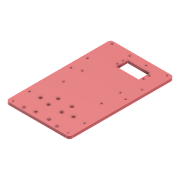
# Autodesk Inventor part: base plate
Saved by Autodesk Inventor 2022 (Build 260153000, 153)
## iProperties
Created: 2024-03-20
Part Number: base plate
Material: Generic
Document SubType Name: Modeling
Designer: david
Density: 1 g/cm^3
Appearance: Smooth - Red
Author: david
Autodesk Inventor part; units mm, degrees
ref_plane "YZ Plane" through (0, 0, 0) normal (1, 0, 0) x (0, 1, 0)
ref_plane "XZ Plane" through (0, 0, 0) normal (0, 1, 0) x (-1, 0, 0)
ref_plane "XY Plane" through (0, 0, 0) normal (0, 0, 1) x (1, 0, 0)
sketch "Sketch1" plane through (0, 0, 0) normal (0, 1, 0) x (-1, 0, 0)
  line L0 (57.5, -190) -> (57.5, -190) construction
  line L1 (-57.5, -190) -> (-57.5, 0) construction
  line L2 (-57.5, 0) -> (57.5, 0)
  line L3 (57.5, 0) -> (57.5, -190) construction
  line L4 (80.5, 0) -> (-80.5, 0) construction
  line L5 (0, -228) -> (0, 38) construction
  line L6 (57.5, -190) -> (-57.5, -190)
  line L7 (-57.5, -190) -> (-57.5, -190) construction
  line L8 (-57.5, 0) -> (57.5, 0)
  line L9 (57.5, 0) -> (57.5, -40)
  line L10 (57.5, -40) -> (-57.5, -40) construction
  line L11 (-57.5, -40) -> (-57.5, 0)
  line L12 (57.5, -40) -> (57.5, -190)
  line L13 (-57.5, -190) -> (-57.5, -40)
  point P0 (0, 0)
  dimension "width" = 115
  dimension "Length" = 190
  dimension "d2" = 115
  dimension "d92" = 40
  constraints: 24 end point, 6 parallel, 4 horizontal, 4 perpendicular, 1 collinear, 1 point on line, 1 symmetric about line, 1 vertical alignment, 1 other
  measures "width" distance of L1.end L2.end
  measures "Length" distance of L1.start L1.end
  measures "d2" distance of L6.end L0.end
  measures "d92" distance between parallel lines of L2 L10
extrude "Base" add sketch "Sketch1" against normal blind 5
sketch "Sketch2" plane through (0, 0, 0) normal (0, 1, 0) x (1, 0, 0)
  line L0 (30, 35) -> (50, 35) construction
  line L1 (50, 35) -> (50, 5) construction
  line L2 (50, 5) -> (30, 5) construction
  line L3 (30, 5) -> (30, 35) construction
  line L4 (0, 228) -> (0, -38) construction
  line L5 (-30, 35) -> (-50, 35) construction
  line L6 (-50, 35) -> (-50, 5) construction
  line L7 (-50, 5) -> (-30, 5) construction
  line L8 (-30, 5) -> (-30, 35) construction
  line L9 (-57.5, 0) -> (57.5, 0) projected
  line L10 (-35, 40) -> (-25, 40) construction
  line L11 (-25, 40) -> (-25, 0) construction
  line L12 (-25, 0) -> (-35, 0) construction
  line L13 (-35, 0) -> (-35, 40) construction
  line L14 (-30, 30) -> (-30, 10) construction
  line L15 (30, 5) -> (30, 35) construction
  line L16 (35, 40) -> (25, 40) construction
  line L17 (25, 40) -> (25, 0) construction
  line L18 (25, 0) -> (35, 0) construction
  line L19 (35, 0) -> (35, 40) construction
  line L20 (30, 30) -> (30, 10) construction
  point P0 (0, 0)
  point P1 (-30, 40)
  point P2 (-30, 20)
  point P3 (-25, 20)
  point P4 (-30, 20)
  point P5 (30, 40)
  point P6 (30, 20)
  point P7 (25, 20)
  point P8 (30, 20)
  dimension "d5" = 20
  dimension "d6" = 30
  dimension "d8" = 5
  dimension "d16" = 10
  dimension "d18" = 20
  dimension "d19" = 10
  dimension "d20" = 50
  constraints: 38 end point, 18 symmetric about line, 8 coincident, 4 midpoint, 4 parallel, 4 point on line, 2 horizontal, 2 perpendicular, 1 horizontal alignment, 1 vertical alignment
  measures "d5" distance of L1.end L2.end
  measures "d6" distance of L0.end L1.end
  measures "d8" distance between parallel lines of L9 L2
  measures "d16" distance of L10.start L10.end
  measures "d18" distance of L14.end L14.start
  measures "d19" vertical distance of L10.end L14.start
  measures "d20" distance between parallel lines of L17 L11
hole "Bearing Holder Mounting Holes" at (30, 0, -35) at (50, 0, -35) at (50, 0, -5) at (-50, 0, -5) at (-30, 0, -35) at (-50, 0, -35) at (-30, 0, -5) at (30, 0, -5) direction (0, -1, 0) diameter 3.4 end through all
fillet "Fillet1" radius 5 4 edges at (57.5, -2.5, 0) (57.5, -2.5, -190) (-57.5, -2.5, -190) (-57.5, -2.5, 0)
sketch "Sketch5" plane through (0, 0, 0) normal (0, 1, 0) x (1, 0, 0)
  line L0 (-34.5, 81.5) -> (34.5, 81.5) construction
  line L1 (34.5, 81.5) -> (34.5, 115.5) construction
  line L2 (34.5, 115.5) -> (-34.5, 115.5) construction
  line L3 (-34.5, 115.5) -> (-34.5, 81.5) construction
  line L4 (-57.5, 0) -> (52.5, 0) projected
  point P0 (0, 0)
  point P1 (-52.2987, 0)
  point P2 (0, 81.5)
  dimension "d41" = 34
  dimension "d42" = 69
  dimension "d43" = 81.5
  constraints: 8 end point, 2 parallel, 1 horizontal, 1 midpoint, 1 perpendicular, 1 vertical alignment
  measures "d41" distance of L2.end L0.start
  measures "d42" distance of L1.end L2.end
  measures "d43" distance between parallel lines of L4 L0
hole "12v Motor Mount Mounting Holes" at (-34.5, 0, -115.5) at (-34.5, 0, -81.5) at (34.5, 0, -81.5) at (34.5, 0, -115.5) direction (0, -1, 0) diameter 3.2 end through all
sketch "Sketch8" plane through (0, 0, 0) normal (0, 1, 0) x (1, 0, 0)
  line L0 (-10, 153.5) -> (30, 153.5)
  line L1 (30, 153.5) -> (30, 173.5)
  line L2 (30, 173.5) -> (-10, 173.5)
  line L3 (-10, 173.5) -> (-10, 153.5)
  line L4 (52.5, 190) -> (-52.5, 190) projected
  line L5 (-57.5, 0) -> (52.5, 0) projected
  point P0 (0, 0)
  point P1 (0, 190)
  dimension "d64" = 20
  dimension "d65" = 40
  dimension "d67" = 10
  dimension "d107" = 153.5
  constraints: 8 end point, 2 parallel, 1 horizontal, 1 midpoint, 1 perpendicular
  measures "d64" distance of L2.end L0.start
  measures "d65" distance of L1.end L2.end
  measures "d67" distance from line of point (0, 190) L3
  measures "d107" distance between parallel lines of L5 L0
extrude "Servo Cutout 2" cut sketch "Sketch8" against normal through all
sketch "Sketch9" plane through (0, 0, 0) normal (0, 1, 0) x (1, 0, 0)
  line L0 (-13.925, 158.5) -> (33.925, 158.5) construction
  line L1 (33.925, 158.5) -> (33.925, 168.5) construction
  line L2 (33.925, 168.5) -> (-13.925, 168.5) construction
  line L3 (-13.925, 168.5) -> (-13.925, 158.5) construction
  line L4 (30, 173.5) -> (30, 153.5) construction
  line L5 (-10, 153.5) -> (-10, 173.5) construction
  point P0 (0, 0)
  point P1 (-10, 163.5)
  point P2 (-13.925, 163.5)
  point P3 (-10, 163.5)
  dimension "d70" = 3.925
  dimension "d71" = 5
  dimension "d72" = 3.925
  constraints: 8 end point, 3 midpoint, 2 parallel, 1 horizontal, 1 horizontal alignment, 1 perpendicular
  measures "d70" distance between parallel lines of L1 L4
  measures "d71" vertical distance of L2.end point (-10, 163.5)
  measures "d72" distance between parallel lines of L5 L3
hole "Servo Mounting Holes 2" at (-13.925, 0, -158.5) at (-13.925, 0, -168.5) at (33.925, 0, -158.5) at (33.925, 0, -168.5) direction (0, -1, 0) diameter 3.4 end through all
sketch "Sketch10" plane through (0, 0, 0) normal (0, 1, 0) x (1, 0, 0)
  circle A0 centre (33.925, 158.5) radius 1.7 construction
  circle A1 centre (-13.925, 158.5) radius 1.7 construction
  circle A2 centre (-13.925, 168.5) radius 1.7 construction
  circle A3 centre (33.925, 168.5) radius 1.7 construction
  line L0 (-10, 153.5) -> (30, 153.5) construction
  line L1 (30, 153.5) -> (30, 173.5) construction
  line L2 (30, 173.5) -> (-10, 173.5) construction
  line L3 (-10, 173.5) -> (-10, 153.5) construction
  circle A4 centre (34.5, 81.5) radius 1.6 construction
  circle A5 centre (-34.5, 115.5) radius 1.6 construction
  circle A6 centre (-34.5, 81.5) radius 1.6 construction
  circle A7 centre (34.5, 115.5) radius 1.6 construction
  arc A8 (52.5, 0) -> (57.5, 5) centre (52.5, 5) ccw construction
  line L4 (52.5, 0) -> (-52.5, 0) construction
  line L5 (-57.5, 5) -> (-57.5, 185) construction
  line L6 (-52.5, 190) -> (52.5, 190) construction
  line L7 (57.5, 185) -> (57.5, 5) construction
  circle A9 centre (-30, 5) radius 1.7 construction
  circle A10 centre (-30, 35) radius 1.7 construction
  circle A11 centre (50, 5) radius 1.7 construction
  circle A12 centre (30, 35) radius 1.7 construction
  circle A13 centre (50, 35) radius 1.7 construction
  circle A14 centre (-50, 5) radius 1.7 construction
  circle A15 centre (-50, 35) radius 1.7 construction
  circle A16 centre (30, 5) radius 1.7 construction
  line L8 (0, 229.4046) -> (0, -39.4422) construction
  arc A17 (-52.5, 190) -> (-57.5, 185) centre (-52.5, 185) ccw projected
  arc A18 (57.5, 185) -> (52.5, 190) centre (52.5, 185) ccw projected
  arc A19 (-57.5, 5) -> (-52.5, 0) centre (-52.5, 5) ccw projected
  point P0 (-50, 185)
  point P1 (50, 185)
  dimension "d93" = 5
  dimension "d94" = 50
  dimension "d111" = 50
  constraints: 1 symmetric about line
  measures "d93" distance from line of L6 point (-50, 185)
  measures "d94" distance from line of L8 point (-50, 185)
  measures "d111" distance from line of A14.centre L8
hole "Extra Holes For Top Plate" at (-50, 0, -185) at (50, 0, -185) direction (0, -1, 0) diameter 3.4 depth 6
sketch "Sketch11" plane through (0, 0, 0) normal (0, 1, 0) x (1, 0, 0)
  line L0 (49.5, 140) -> (49.5, 110) construction
  line L1 (52.5, 190) -> (-52.5, 190) construction
  line L2 (0, 228) -> (0, -38) projected
  line L3 (-49.5, 140) -> (-49.5, 110) construction
  line L4 (15, 182) -> (-15, 182)
  line L5 (57.5, 5) -> (57.5, 185) projected
  point P0 (0, 0)
  point P1 (0, 182)
  point P2 (0, 190)
  dimension "d95" = 50
  dimension "d96" = 30
  dimension "d108" = 30
  dimension "d109" = 8
  dimension "d110" = 8
  constraints: 6 coincident, 6 end point, 4 symmetric about line, 2 midpoint, 1 horizontal, 1 parallel, 1 vertical alignment
  measures "d95" distance from line of L1 L0.start
  measures "d96" distance of L0.start L0.end
  measures "d108" distance of L4.start L4.end
  measures "d109" distance between parallel lines of L1 L4
  measures "d110" distance between parallel lines of L5 L0
hole "Ultrasonic Sensor Mounting Holes" at (49.5, 0, -140) at (49.5, 0, -110) at (-49.5, 0, -110) at (-49.5, 0, -140) at (-15, 0, -182) at (15, 0, -182) direction (0, -1, 0) diameter 3.4 depth 6
thicken "Thicken2" operation add thickness 0.45 both sides no extend neighbours yes toward (-1, 0, 0) faces at (-10, -1.6667, -166.8333) (16.6667, -3.3333, -173.5) (3.3333, -1.6667, -153.5) (30, -1.6667, -160.1667)
sketch "Sketch12" plane through (0, 0, 0) normal (0, 1, 0) x (1, 0, 0)
  circle A0 centre (30, 35) radius 1.7 construction
  circle A1 centre (30, 5) radius 1.7 construction
  line L0 (30, 35) -> (30, 5) construction
  line L1 (-12, 31.5) -> (12, 31.5)
  line L2 (12, 31.5) -> (12, 8.5)
  line L3 (12, 8.5) -> (-12, 8.5)
  line L4 (-12, 8.5) -> (-12, 31.5)
  line L5 (-12, 31.5) -> (12, 8.5) construction
  line L6 (12, 31.5) -> (-12, 8.5) construction
  point P0 (0, 0)
  point P1 (12, 20)
  point P2 (30, 20)
  point P3 (0, 8.5)
  point P4 (-12, 31.5)
  point P5 (12, 31.5)
  point P6 (0, 20)
  point P7 (0, 20)
  point P8 (0, 20)
  dimension "d121" = 23
  dimension "d122" = 24
  constraints: 14 end point, 5 midpoint, 2 coincident, 2 horizontal alignment, 2 parallel, 2 vertical alignment, 1 horizontal, 1 perpendicular, 1 vertical
  measures "d121" distance of L1.end L2.end
  measures "d122" distance of L1.start L1.end
hole "Differential Stopper Mounting Holes" at (-12, 0, -31.5) at (12, 0, -31.5) at (-12, 0, -8.5) at (12, 0, -8.5) direction (0, -1, 0) diameter 3.4 end through all counterbore diameter 6 counterbore depth 2
sketch "Sketch13" plane through (0, 0, 0) normal (0, -1, 0) x (1, 0, 0)
  line L0 (-12.5, -49.5) -> (12.5, -49.5)
  line L1 (52.5, 0) -> (-52.5, 0) projected
  point P0 (0, 0)
  point P1 (0, -49.5)
  point P2 (-57.5, 0)
  dimension "d123" = 25
  dimension "d124" = 49.5
  constraints: 2 coincident, 2 end point, 1 horizontal, 1 midpoint, 1 vertical alignment
  measures "d123" distance of L0.start L0.end
  measures "d124" distance between parallel lines of L1 L0
hole "Driver Gear Stopper Mounting Holes" at (-12.5, 0, -49.5) at (12.5, 0, -49.5) direction (0, -1, 0) diameter 3.4 end through all counterbore diameter 6 counterbore depth 2
sketch "Sketch15" plane through (0, 0, 0) normal (0, 1, 0) x (1, 0, 0)
  circle A0 centre (-30, 35) radius 1.7 projected
  circle A1 centre (-30, 5) radius 1.7 projected
  circle A2 centre (30, 35) radius 1.7 projected
  circle A3 centre (30, 5) radius 1.7 projected
  point P0 (0, 0)
  constraints: 4 coincident
hole "CounterBore for Bearing Holder Mounting Holes" at (-30, 0, -35) at (-30, 0, -5) at (30, 0, -35) at (30, 0, -5) direction (0, -1, 0) diameter 6 depth 2
equation "\"d2\" = width"
equation "\"d9\" = HoleDia"
equation "\"d72\" = d70"
equation "\"d73\" = HoleDia"
equation "\"d94\" = d111"
equation "\"d84\" = HoleDia"
equation "\"d109\" = d97"
equation "\"d98\" = HoleDia"
equation "\"d114\" = HoleDia"
equation "\"d125\" = HoleDia"
equation "\"HoleDia\" = 3.4"
equation "\"d97\" = 8"
body "Solid1"
